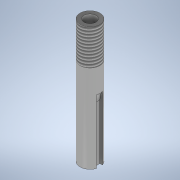
# Autodesk Inventor part: Tornillo deslizante
Saved by Autodesk Inventor 2020 (Build 240168000, 168)
## iProperties
Created: 2020-09-17
Part Number: Tornillo deslizante
Material: Steel AISI 1045 HV HR
Document SubType Name: Modeling
Designer: aaron
Density: 7.85 g/cm^3
Appearance: Steel Doors - Painted White
Author: aaron
Autodesk Inventor part; units mm, degrees
ref_plane "YZ Plane" through (0, 0, 0) normal (1, 0, 0) x (0, 1, 0)
ref_plane "XZ Plane" through (0, 0, 0) normal (0, 1, 0) x (-1, 0, 0)
ref_plane "XY Plane" through (0, 0, 0) normal (0, 0, 1) x (1, 0, 0)
sketch "Sketch1" plane through (0, 0, 0) normal (0, 1, 0) x (-1, 0, 0)
  circle A0 centre (0, 0) radius 7.9248
  dimension "d0" = 15.8496
  constraints: 1 centre point, 1 coincident
  measures "d0" diameter of A0
extrude "Extrusion1" add sketch "Sketch1" along normal blind 98.425
sketch "Sketch2" plane through (0, 98.425, 0) normal (0, 1, 0) x (1, 0, 0)
  circle A0 centre (0, 0) radius 4.7498
  dimension "d3" = 9.4996
  constraints: 1 centre point, 1 coincident
  measures "d3" diameter of A0
extrude "Extrusion2" cut sketch "Sketch2" against normal blind 50.8
thread "Thread1" size "5/8-11 UNC" class "2A" standard "ANSI Unified Screw Threads" length 28.575
sketch "Sketch3" plane through (0, 0, 0) normal (0, -1, 0) x (1, 0, 0)
  line L0 (-11.0947, 0) -> (11.0947, 0) projected
  circle A0 centre (0, 0) radius 7.9248 projected
  line L1 (7.9248, 0) -> (5.5435, 0) construction
  line L2 (5.5435, 0) -> (5.5435, -2.3813)
  line L3 (5.5435, -2.3813) -> (7.5586, -2.3813)
  line L4 (5.5435, 0) -> (5.5435, 2.3813)
  line L5 (5.5435, 2.3813) -> (7.5586, 2.3813)
  dimension "d8" = 2.3813
  dimension "d9" = 2.3813
  constraints: 10 end point, 2 point on circle, 2 point on line, 2 symmetric about line, 1 horizontal, 1 vertical
  measures "d8" distance of L1.end L1.start
  measures "d9" distance between parallel lines of L0 L3
extrude "Extrusion3" cut sketch "Sketch3" against normal blind 50.8 contours L4 L5 A0 L0 | L0 A0 L3 L2 picked at (6.2828, 1.3275) picked at (6.2828, -1.3275)
fillet "Fillet1" radius 11.1125 1 edges at (5.5435, 50.8, 0)
body "Solid1"
